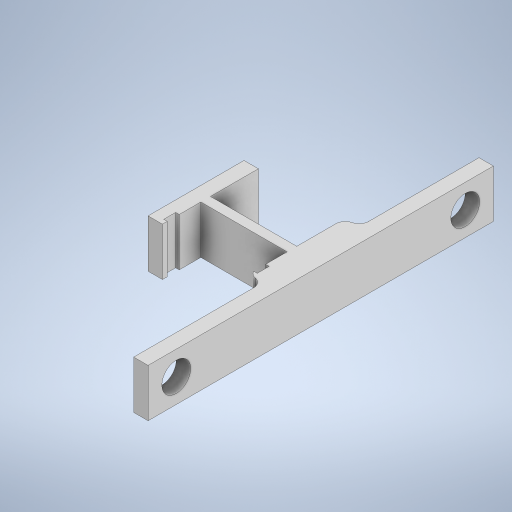
# Autodesk Inventor part: CO-1-01-stepperControllerMount
Saved by Autodesk Inventor 2024 (Build 280153000, 153)
## iProperties
Created: 2023-11-20
Part Number: CO-1-01-stepperControllerMount
Material: Generic
Document SubType Name: Modeling
Designer: t205b
Density: 1 g/cm^3
Appearance: Default
Author: t205b
Autodesk Inventor part; units mm, degrees
ref_plane "YZ Plane" through (0, 0, 0) normal (1, 0, 0) x (0, 1, 0)
ref_plane "XZ Plane" through (0, 0, 0) normal (0, 1, 0) x (-1, 0, 0)
ref_plane "XY Plane" through (0, 0, 0) normal (0, 0, 1) x (1, 0, 0)
sketch "Sketch1" plane through (0, 0, 0) normal (0, 1, 0) x (-1, 0, 0)
  line L0 (-3.0388, 7.0833) -> (-6.0388, 7.0833)
  line L1 (-6.0388, 7.0833) -> (-6.0388, -12.9167)
  line L2 (-6.0388, -12.9167) -> (-3.0388, -12.9167)
  line L3 (-3.0388, -12.9167) -> (-3.0388, -2.9167)
  line L4 (-3.0388, -2.9167) -> (14.9612, -2.9167)
  line L5 (14.9612, -12.9167) -> (17.9612, -12.9167)
  line L6 (17.9612, -12.9167) -> (17.9612, 7.0833)
  line L7 (17.9612, 7.0833) -> (14.9612, 7.0833)
  line L8 (14.9612, 7.0833) -> (14.9612, 6.0833)
  line L9 (14.9612, 6.0833) -> (15.7112, 6.0833)
  line L10 (15.7112, 6.0833) -> (15.7112, 3.5833)
  line L11 (15.7112, 3.5833) -> (14.9612, 3.5833)
  line L12 (14.9612, 3.5833) -> (14.9612, -0.9167)
  line L13 (14.9612, -0.9167) -> (-3.0388, -0.9167)
  line L14 (-3.0388, -0.9167) -> (-3.0388, 3.5833)
  line L15 (-3.7888, 3.5833) -> (-3.7888, 6.0833)
  line L16 (-3.7888, 6.0833) -> (-3.0388, 6.0833)
  line L17 (-3.0388, 3.5833) -> (-3.7888, 3.5833)
  line L18 (-3.0388, 6.0833) -> (-3.0388, 7.0833)
  line L19 (14.9612, -12.9167) -> (14.9612, -2.9167)
  line L20 (-6.0388, 7.0833) -> (-6.0388, 34.0833)
  line L21 (-6.0388, 34.0833) -> (-9.0388, 34.0833)
  line L22 (-9.0388, 34.0833) -> (-9.0388, -37.9167)
  line L23 (-9.0388, -37.9167) -> (-6.0388, -37.9167)
  line L24 (-6.0388, -37.9167) -> (-6.0388, -12.9167)
  point P0 (0, 0)
  point P1 (14.9612, 1.3333)
  dimension "d0" = 2.5
  dimension "d1" = 3
  dimension "d2" = 3
  dimension "d3" = 10
  dimension "d4" = 10
  dimension "d5" = 2
  dimension "d6" = 3
  dimension "d8" = 1
  dimension "d9" = 8
  dimension "d11" = 0.75
  dimension "d12" = 0.75
  dimension "d13" = 3
  dimension "d16" = 18
  dimension "d17" = 3
  dimension "d18" = 72
  dimension "d19" = 35
  constraints: 50 end point, 16 perpendicular, 11 point on line, 2 horizontal, 2 vertical, 1 midpoint, 1 other
  measures "d0" distance between parallel lines of L16 L17
  measures "d1" distance between parallel lines of L3 L1
  measures "d2" distance between parallel lines of L14 L1
  measures "d3" distance between parallel lines of L4 L2
  measures "d4" distance between parallel lines of L4 L5
  measures "d5" distance between parallel lines of L13 L4
  measures "d6" distance between parallel lines of L6 L12
  measures "d8" distance between parallel lines of L0 L16
  measures "d9" distance between parallel lines of L0 L13
  measures "d11" distance between parallel lines of L14 L15
  measures "d12" distance between parallel lines of L10 L12
  measures "d13" distance between parallel lines of L6 L19
  measures "d16" distance from line of point (14.961, 1.333) L14
  measures "d17" distance between parallel lines of L20 L22
  measures "d18" distance between parallel lines of L23 L21
  measures "d19" distance between parallel lines of L4 L23
extrude "Extrusion1" add sketch "Sketch1" along normal blind 10
fillet "Fillet1" radius 2 4 edges at (6.0388, 5, 7.0833) (6.0388, 5, -12.9167) (3.0388, 5, -12.9167) (3.0388, 5, 7.0833)
sketch "Sketch2" plane through (6.0388, 0, 34.0833) normal (-1, 0, 0) x (0, 0, 1)
  circle A0 centre (-5.875, 5) radius 3
  circle A1 centre (-66.125, 5) radius 3
  line L0 (-72, 0) -> (-49, 0) projected
  line L1 (-72, 10) -> (-49, 10) projected
  line L2 (-25, 10) -> (0, 10) projected
  line L3 (0, 0) -> (0, 10) projected
  line L4 (-72, 0) -> (-72, 10) projected
  point P0 (-34.0833, 0)
  dimension "d21" = 6
  dimension "d22" = 6
  dimension "d23" = 10
  dimension "d24" = 5
  dimension "d25" = 5
  dimension "d26" = 60.25
  dimension "d27" = 72
  dimension "d28" = 5.875
  constraints: 2 centre point
  measures "d21" diameter of A0
  measures "d22" diameter of A1
  measures "d23" distance between parallel lines of L0 L1
  measures "d24" distance from line of A1.centre L1
  measures "d25" distance from line of A0.centre L2
  measures "d26" distance of A0.centre A1.centre
  measures "d27" distance between parallel lines of L3 L4
  measures "d28" distance from line of A0.centre L3
extrude "Extrusion2" cut sketch "Sketch2" against normal through all
equation "\"d2\" = d1"
equation "\"d4\" = d3"
equation "\"d6\" = d2"
equation "\"d12\" = d11"
equation "\"d13\" = d1"
equation "\"d19\" = -0.5 * d5 + 0.5 * d18"
equation "\"d24\" = 0.5 * d23"
equation "\"d25\" = 0.5 * d23"
equation "\"d28\" = -0.5 * d26 + 0.5 * d27"
body "Solid1"
